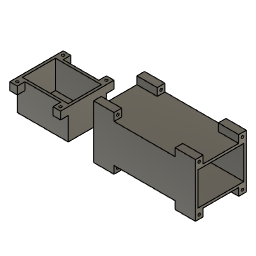
batteripakkeholder v1 (Autodesk Fusion 360 design; units mm, degrees)
Autodesk Fusion 360 part; units mm, degrees
sketch "Sketch1" plane through (0, 0, 0) normal (0, 0, 1) x (1, 0, 0)
  line L0 (0, 0) -> (330, 0)
  line L1 (330, 0) -> (330, 100)
  line L2 (330, 100) -> (0, 100)
  line L3 (0, 100) -> (0, 0)
  dimension "d1" = 330
  dimension "d2" = 100
  constraint horizontal L0
  constraint vertical L1
  constraint horizontal L2
  constraint vertical L3
  constraint coincident L0.start L3.end
  measures "d1" distance of L0.start L0.end
  measures "d2" distance of L0.start L2.end
sketch "Sketch2" plane through (0, 0, 0) normal (0, 0, 1) x (1, 0, 0)
  line L0 (0, 0) -> (200, 0)
  line L1 (200, 0) -> (200, 100)
  line L2 (200, 100) -> (0, 100)
  line L3 (0, 100) -> (0, 0)
  dimension "d7" = 200
  dimension "d8" = 100
  constraint horizontal L0
  constraint vertical L1
  constraint horizontal L2
  constraint vertical L3
  constraint coincident L0.start L3.end
  measures "d7" distance of L0.start L0.end
  measures "d8" distance of L0.start L2.end
extrude "Extrude3" add sketch "Sketch2" along normal blind 5 makes body 1
sketch "Sketch3" plane through (0, 0, 5) normal (0, 0, 1) x (-1, 0, 0)
  line L0 (0, -100) -> (0, 0)
  line L1 (0, 0) -> (-200, 0)
  line L2 (-200, 0) -> (-200, -100)
  line L3 (-200, -100) -> (0, -100)
  line L4 (0, 0) -> (-200, 0)
  line L5 (-200, 0) -> (-200, -5)
  line L6 (-200, -5) -> (0, -5)
  line L7 (0, -5) -> (0, 0)
  line L8 (0, -100) -> (-200, -100)
  line L9 (-200, -100) -> (-200, -95)
  line L10 (-200, -95) -> (0, -95)
  line L11 (0, -95) -> (0, -100)
  dimension "d11" = 5
  dimension "d12" = 5
  constraint horizontal L4
  constraint vertical L5
  constraint horizontal L6
  constraint vertical L7
  constraint coincident L0.end L1.start
  constraint horizontal L8
  constraint vertical L9
  constraint horizontal L10
  constraint vertical L11
  constraint coincident L0.start L3.end
  measures "d11" distance of L0.end L6.end
  measures "d12" distance of L0.start L10.end
extrude "Extrude4" add sketch "Sketch3" along normal blind 65 contours L0 L2 L3 L8 L9 L10 L11 | L0 L1 L2 L4 L5 L6 L7 bodies 1
sketch "Sketch4" plane through (0, 0, 70) normal (0, 0, 1) x (-1, 0, 0)
  line L0 (0, -5) -> (0, 0)
  line L1 (0, 0) -> (-200, 0)
  line L2 (-200, 0) -> (-200, -5)
  line L3 (-200, -5) -> (0, -5)
  line L4 (0, 0) -> (-200, 0)
  line L5 (-200, 0) -> (-200, -100)
  line L6 (-200, -100) -> (0, -100)
  line L7 (0, -100) -> (0, 0)
  constraint horizontal L4
  constraint vertical L5
  constraint horizontal L6
  constraint vertical L7
  constraint coincident L0.end L1.start
extrude "Extrude5" add sketch "Sketch4" along normal blind 5 bodies 1
sketch "Sketch5" plane through (0, 0, 0) normal (0, 0, -1) x (1, 0, 0)
  line L0 (0, 0) -> (0, -100)
  line L1 (0, -100) -> (200, -100)
  line L2 (200, -100) -> (200, 0)
  line L3 (200, 0) -> (0, 0)
  line L4 (200, 0) -> (160, 0)
  line L5 (160, 0) -> (160, -15)
  line L6 (160, -15) -> (200, -15)
  line L7 (200, -15) -> (200, 0)
  line L8 (200, -100) -> (160, -100)
  line L9 (160, -100) -> (160, -85)
  line L10 (160, -85) -> (200, -85)
  line L11 (200, -85) -> (200, -100)
  line L12 (0, -100) -> (40, -100)
  line L13 (40, -100) -> (40, -85)
  line L14 (40, -85) -> (0, -85)
  line L15 (0, -85) -> (0, -100)
  line L16 (0, 0) -> (40, 0)
  line L17 (40, 0) -> (40, -15)
  line L18 (40, -15) -> (0, -15)
  line L19 (0, -15) -> (0, 0)
  dimension "d17" = 15
  dimension "d18" = 40
  dimension "d19" = 15
  dimension "d20" = 15
  dimension "d21" = 40
  dimension "d22" = 15
  constraint horizontal L4
  constraint vertical L5
  constraint horizontal L6
  constraint vertical L7
  constraint coincident L2.end L3.start
  constraint horizontal L8
  constraint vertical L9
  constraint horizontal L10
  constraint vertical L11
  constraint coincident L1.end L2.start
  constraint horizontal L12
  constraint vertical L13
  constraint horizontal L14
  constraint vertical L15
  constraint coincident L0.end L1.start
  constraint horizontal L16
  constraint vertical L17
  constraint horizontal L18
  constraint vertical L19
  constraint coincident L0.start L3.end
  measures "d17" distance of L2.end L6.end
  measures "d18" distance of L1.end L8.end
  measures "d19" distance of L1.end L10.end
  measures "d20" distance of L0.end L14.end
  measures "d21" distance of L0.start L16.end
  measures "d22" distance of L0.start L18.end
extrude "Extrude6" add sketch "Sketch5" along normal blind 15 contours L0 L3 L16 L17 L18 L19 | L0 L1 L12 L13 L14 L15 | L2 L3 L4 L5 L6 L7 | L1 L2 L8 L9 L10 L11 bodies 1
sketch "Sketch6" plane through (0, 0, 75) normal (0, 0, 1) x (-1, 0, 0)
  line L0 (0, -100) -> (0, 0)
  line L1 (0, 0) -> (-200, 0)
  line L2 (-200, 0) -> (-200, -100)
  line L3 (-200, -100) -> (0, -100)
  line L4 (-200, -100) -> (-160, -100)
  line L5 (-160, -100) -> (-160, -85)
  line L6 (-160, -85) -> (-200, -85)
  line L7 (-200, -85) -> (-200, -100)
  line L8 (-200, 0) -> (-160, 0)
  line L9 (-160, 0) -> (-160, -15)
  line L10 (-160, -15) -> (-200, -15)
  line L11 (-200, -15) -> (-200, 0)
  line L12 (0, 0) -> (-40, 0)
  line L13 (-40, 0) -> (-40, -15)
  line L14 (-40, -15) -> (0, -15)
  line L15 (0, -15) -> (0, 0)
  line L16 (0, -100) -> (-40, -100)
  line L17 (-40, -100) -> (-40, -85)
  line L18 (-40, -85) -> (0, -85)
  line L19 (0, -85) -> (0, -100)
  dimension "d25" = 40
  dimension "d26" = 15
  dimension "d27" = 15
  dimension "d28" = 15
  dimension "d29" = 40
  dimension "d30" = 15
  constraint horizontal L4
  constraint vertical L5
  constraint horizontal L6
  constraint vertical L7
  constraint coincident L2.end L3.start
  constraint horizontal L8
  constraint vertical L9
  constraint horizontal L10
  constraint vertical L11
  constraint coincident L1.end L2.start
  constraint horizontal L12
  constraint vertical L13
  constraint horizontal L14
  constraint vertical L15
  constraint coincident L0.end L1.start
  constraint horizontal L16
  constraint vertical L17
  constraint horizontal L18
  constraint vertical L19
  constraint coincident L0.start L3.end
  measures "d25" distance of L2.end L4.end
  measures "d26" distance of L2.end L6.end
  measures "d27" distance of L1.end L10.end
  measures "d28" distance of L0.end L14.end
  measures "d29" distance of L0.start L16.end
  measures "d30" distance of L0.start L18.end
extrude "Extrude7" add sketch "Sketch6" along normal blind 15 contours L0 L3 L16 L17 L18 L19 | L0 L1 L12 L13 L14 L15 | L2 L3 L4 L5 L6 L7 | L1 L2 L8 L9 L10 L11 bodies 1
hole "Hole1" at (200, 92.5, 82.5) direction (-1, 0, 0) diameter 5 depth 500 tip angle 118 bodies 1
hole "Hole2" at (200, 7.5, 82.5) direction (-1, 0, 0) diameter 5 depth 500 tip angle 118 bodies 1
hole "Hole3" at (200, 92.5, -7.5) direction (-1, 0, 0) diameter 5 depth 500 tip angle 118 bodies 1
hole "Hole4" at (200, 7.5, -7.5) direction (-1, 0, 0) diameter 5 depth 500 tip angle 118 bodies 1
sketch "Sketch7" plane through (0, 0, 0) normal (0, 0, 1) x (1, 0, 0)
  line L0 (-50, 0) -> (-140, 0)
  line L1 (-140, 0) -> (-140, 65)
  line L2 (-140, 65) -> (-50, 65)
  line L3 (-50, 65) -> (-50, 0)
  line L4 (-45, -5) -> (-145, -5)
  line L5 (-145, -5) -> (-145, 70)
  line L6 (-145, 70) -> (-45, 70)
  line L7 (-45, 70) -> (-45, -5)
  dimension "d53" = 90
  dimension "d54" = 65
  constraint horizontal L0
  constraint vertical L1
  constraint horizontal L2
  constraint vertical L3
  constraint horizontal L4
  constraint vertical L5
  constraint horizontal L6
  constraint vertical L7
  measures "d53" distance of L0.start L0.end
  measures "d54" distance of L0.start L2.end
extrude "Extrude1" add sketch "Sketch7" along normal blind 5 separate body contours L0 L1 L2 L3 | L4 L5 L6 L7 makes body 2 in component "Component"
sketch "Sketch8" plane through (0, 0, 5) normal (0, 0, 1) x (-1, 0, 0)
  line L0 (45, -70) -> (145, -70)
  line L1 (145, -70) -> (145, 5)
  line L2 (145, 5) -> (45, 5)
  line L3 (45, 5) -> (45, -70)
  line L4 (140, -65) -> (50, -65)
  line L5 (50, -65) -> (50, 0)
  line L6 (50, 0) -> (140, 0)
  line L7 (140, 0) -> (140, -65)
  constraint horizontal L4
  constraint vertical L5
  constraint horizontal L6
  constraint vertical L7
extrude "Extrude2" add sketch "Sketch8" along normal blind 55 bodies 2 in component "Component"
sketch "Sketch9" plane through (0, -5, 0) normal (0, -1, 0) x (1, 0, 0)
  line L0 (-145, 0) -> (-45, 0)
  line L1 (-45, 0) -> (-45, 60)
  line L2 (-45, 60) -> (-145, 60)
  line L3 (-145, 60) -> (-145, 0)
  line L4 (-145, 60) -> (-130, 60)
  line L5 (-130, 60) -> (-130, 45)
  line L6 (-130, 45) -> (-145, 45)
  line L7 (-145, 45) -> (-145, 60)
  line L8 (-45, 60) -> (-60, 60)
  line L9 (-60, 60) -> (-60, 45)
  line L10 (-60, 45) -> (-45, 45)
  line L11 (-45, 45) -> (-45, 60)
  constraint horizontal L4
  constraint vertical L5
  constraint horizontal L6
  constraint vertical L7
  constraint coincident L2.end L3.start
  constraint horizontal L8
  constraint vertical L9
  constraint horizontal L10
  constraint vertical L11
  constraint coincident L1.end L2.start
extrude "Extrude3'" add sketch "Sketch9" along normal blind 15 contours L2 L3 L4 L5 L6 L7 | L1 L2 L8 L9 L10 L11 bodies 2 in component "Component"
sketch "Sketch10" plane through (0, 70, 0) normal (0, 1, 0) x (-1, 0, 0)
  line L0 (45, 0) -> (145, 0)
  line L1 (145, 0) -> (145, 60)
  line L2 (145, 60) -> (45, 60)
  line L3 (45, 60) -> (45, 0)
  line L4 (45, 60) -> (60, 60)
  line L5 (60, 60) -> (60, 45)
  line L6 (60, 45) -> (45, 45)
  line L7 (45, 45) -> (45, 60)
  line L8 (145, 60) -> (130, 60)
  line L9 (130, 60) -> (130, 45)
  line L10 (130, 45) -> (145, 45)
  line L11 (145, 45) -> (145, 60)
  dimension "d61" = 15
  dimension "d62" = 15
  dimension "d63" = 15
  dimension "d64" = 15
  constraint horizontal L4
  constraint vertical L5
  constraint horizontal L6
  constraint vertical L7
  constraint coincident L2.end L3.start
  constraint horizontal L8
  constraint vertical L9
  constraint horizontal L10
  constraint vertical L11
  constraint coincident L1.end L2.start
  measures "d61" distance of L2.end L4.end
  measures "d62" distance of L2.end L6.end
  measures "d63" distance of L1.end L8.end
  measures "d64" distance of L1.end L10.end
extrude "Extrude4'" add sketch "Sketch10" along normal blind 15 contours L2 L3 L4 L5 L6 L7 | L1 L2 L8 L9 L10 L11 bodies 2 in component "Component"
hole "Hole1'" at (-137.5, 77.5, 60) direction (0, 0, -1) diameter 5 depth 500 tip angle 118 bodies 2 in component "Component"
hole "Hole2'" at (-52.5, 77.5, 60) direction (0, 0, -1) diameter 5 depth 500 tip angle 118 bodies 2 in component "Component"
hole "Hole3'" at (-137.5, -12.5, 60) direction (0, 0, -1) diameter 5 depth 500 tip angle 118 bodies 2 in component "Component"
hole "Hole4'" at (-52.5, -12.5, 60) direction (0, 0, -1) diameter 5 depth 500 tip angle 118 bodies 2 in component "Component"
component "Component" placed x (1, 0, 0) y (0, 1, 0) z (0, 0, 1) at (0, 0, 0)
